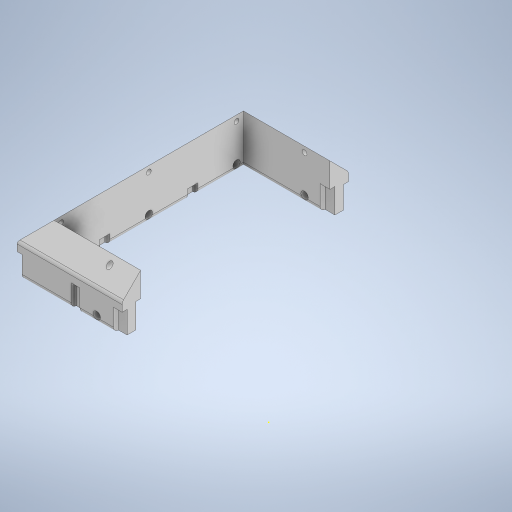
# Autodesk Inventor part: Palm_FingerAttachment
Saved by Autodesk Inventor 2023 (Build 270158000, 158)
## iProperties
Created: 2023-04-19
Part Number: Palm_FingerAttachment
Material: Generic
Document SubType Name: Modeling
Designer: 1senadi
Density: 1 g/cm^3
Appearance: Default
Author: 1senadi
Autodesk Inventor part; units mm, degrees
ref_plane "YZ Plane" through (0, 0, 0) normal (1, 0, 0) x (0, 1, 0)
ref_plane "XZ Plane" through (0, 0, 0) normal (0, 1, 0) x (-1, 0, 0)
ref_plane "XY Plane" through (0, 0, 0) normal (0, 0, 1) x (1, 0, 0)
sketch "Sketch1" plane through (0, 0, 0) normal (0, 1, 0) x (-1, 0, 0)
  line L0 (0, 0) -> (102, 0)
  line L1 (102, 0) -> (102, 91.8)
  line L2 (102, 91.8) -> (0, 91.8)
  line L3 (0, 91.8) -> (0, 0)
  line L4 (94.5, 84.3) -> (94.5, 7.5)
  line L5 (94.5, 7.5) -> (7.5, 7.5)
  line L6 (7.5, 7.5) -> (7.5, 84.3)
  line L7 (7.5, 84.3) -> (94.5, 84.3)
  dimension "d0" = 102
  dimension "d1" = 91.8
  dimension "d2" = 7.5
  constraints: 16 end point, 4 parallel, 2 perpendicular, 1 horizontal, 3 other
  measures "d0" distance of L2.end L1.end
  measures "d1" distance of L1.end L0.end
  measures "d2" distance between parallel lines of L1 L4
extrude "Extrusion1" add sketch "Sketch1" along normal blind 20
sketch "Sketch2" plane through (-102, 0, 0) normal (-1, 0, 0) x (0, 0, 1)
  line L0 (0, 0) -> (0, 9)
  line L1 (0, 0) -> (0, 20) projected
  line L2 (0, 9) -> (3.5, 9)
  line L3 (3.5, 9) -> (3.5, 0)
  line L4 (91.8, 0) -> (0, 0) projected
  line L5 (0, 0) -> (3.5, 0)
  line L6 (3.5, 0) -> (17.1, 0)
  line L7 (17.1, 0) -> (17.1, 9)
  line L8 (17.1, 9) -> (20.6, 9)
  line L9 (20.6, 9) -> (20.6, 0)
  line L10 (17.1, 0) -> (20.6, 0)
  line L11 (56.2, 9) -> (56.2, 0)
  line L12 (52.7, 9) -> (56.2, 9)
  line L13 (52.7, 0) -> (52.7, 9)
  line L14 (52.7, 0) -> (56.2, 0)
  line L15 (39.1, 0) -> (52.7, 0)
  line L16 (39.1, 9) -> (39.1, 0)
  line L17 (35.6, 9) -> (39.1, 9)
  line L18 (35.6, 0) -> (35.6, 9)
  line L19 (35.6, 0) -> (39.1, 0)
  line L20 (91.8, 9) -> (91.8, 0)
  line L21 (88.3, 9) -> (91.8, 9)
  line L22 (88.3, 0) -> (88.3, 9)
  line L23 (88.3, 0) -> (91.8, 0)
  line L24 (74.7, 0) -> (88.3, 0)
  line L25 (74.7, 9) -> (74.7, 0)
  line L26 (71.2, 9) -> (74.7, 9)
  line L27 (71.2, 0) -> (71.2, 9)
  line L28 (71.2, 0) -> (74.7, 0)
  point P0 (88.3, 0)
  point P1 (74.7, 0)
  point P2 (52.7, 0)
  point P3 (39.1, 0)
  dimension "d5" = 9
  dimension "d6" = 3.5
  dimension "d7" = 13.6
  dimension "d8" = 9
  dimension "d9" = 3.5
  dimension "d12" = 35.6
  constraints: 54 end point, 6 perpendicular, 4 point on line, 1 collinear, 1 horizontal, 34 other
  measures "d5" distance of L0.start L0.end
  measures "d6" distance of L0.end L2.end
  measures "d7" distance of L3.end L6.end
  measures "d8" distance of L6.end L7.end
  measures "d9" distance of L7.end L8.end
  measures "d12" distance of L8.end L11.start
extrude "Extrusion2" cut sketch "Sketch2" against normal blind 2
sketch "Sketch3" plane through (-102, 20, 91.8) normal (0, 0, 1) x (1, 0, 0)
  point P0 (102, -20)
sketch "Sketch4" plane through (-102, 20, 91.8) normal (0, 0, 1) x (1, 0, 0)
  line L0 (2, -20) -> (0, -20) projected
  line L1 (2, -20) -> (22, -20)
  line L2 (7.5, -20) -> (94.5, -20) projected
  line L3 (22, -20) -> (22, -11)
  line L4 (22, -11) -> (25.5, -11)
  line L5 (25.5, -11) -> (25.5, -20)
  line L6 (22, -20) -> (25.5, -20)
  line L7 (25.5, -20) -> (39.1, -20)
  line L8 (39.1, -20) -> (39.1, -11)
  line L9 (39.1, -11) -> (42.6, -11)
  line L10 (42.6, -11) -> (42.6, -20)
  line L11 (42.6, -20) -> (39.1, -20)
  point P0 (102, -20)
  dimension "d19" = 20
  dimension "d20" = 9
  dimension "d21" = 3.5
  dimension "d22" = 13.6
  dimension "d23" = 9
  dimension "d24" = 3.5
  constraints: 20 end point, 6 point on line, 3 perpendicular, 2 collinear, 1 vertical
  measures "d19" distance of L0.start L1.end
  measures "d20" distance of L1.end L3.end
  measures "d21" distance of L3.end L4.end
  measures "d22" distance of L5.end L7.end
  measures "d23" distance of L7.end L8.end
  measures "d24" distance of L8.end L9.end
extrude "Extrusion3" cut sketch "Sketch4" against normal blind 2
ref_plane "Work Plane1" through (-102, 0, 45.9) normal (0, 0, 1) x (1, 0, 0)
sketch "Sketch5" plane through (0, 0, 0) normal (0, -1, 0) x (1, 0, 0)
  line L0 (0, 0) -> (-100, 0) projected
  line L1 (0, 91.8) -> (0, 0) projected
  line L2 (-59.4, 91.8) -> (0, 91.8) projected
  line L3 (-59.4, 91.8) -> (-59.4, 89.8) projected
  line L4 (-59.4, 89.8) -> (-62.9, 89.8) projected
  line L5 (-62.9, 89.8) -> (-62.9, 91.8) projected
  line L6 (-76.5, 91.8) -> (-62.9, 91.8) projected
  line L7 (-76.5, 91.8) -> (-76.5, 89.8) projected
  line L8 (-76.5, 89.8) -> (-80, 89.8) projected
  line L9 (-80, 89.8) -> (-80, 91.8) projected
  line L10 (-100, 91.8) -> (-80, 91.8) projected
  line L11 (-100, 91.8) -> (-100, 88.3) projected
  line L12 (-100, 88.3) -> (-102, 88.3) projected
  line L13 (-102, 74.7) -> (-102, 88.3) projected
  line L14 (-102, 74.7) -> (-100, 74.7) projected
  line L15 (-100, 74.7) -> (-100, 71.2) projected
  line L16 (-100, 71.2) -> (-102, 71.2) projected
  line L17 (-102, 56.2) -> (-102, 71.2) projected
  line L18 (-102, 56.2) -> (-100, 56.2) projected
  line L19 (-100, 56.2) -> (-100, 52.7) projected
  line L20 (-100, 52.7) -> (-102, 52.7) projected
  line L21 (-102, 39.1) -> (-102, 52.7) projected
  line L22 (-102, 39.1) -> (-100, 39.1) projected
  line L23 (-100, 39.1) -> (-100, 35.6) projected
  line L24 (-100, 35.6) -> (-102, 35.6) projected
  line L25 (-102, 20.6) -> (-102, 35.6) projected
  line L26 (-102, 20.6) -> (-100, 20.6) projected
  line L27 (-100, 20.6) -> (-100, 17.1) projected
  line L28 (-100, 17.1) -> (-102, 17.1) projected
  line L29 (-102, 3.5) -> (-102, 17.1) projected
  line L30 (-102, 3.5) -> (-100, 3.5) projected
  line L31 (-100, 3.5) -> (-100, 0) projected
  line L32 (-94.5, 84.3) -> (-94.5, 7.5) projected
  line L33 (-7.5, 84.3) -> (-94.5, 84.3) projected
  line L34 (-7.5, 7.5) -> (-7.5, 84.3) projected
  line L35 (-94.5, 7.5) -> (-7.5, 7.5) projected
  line L36 (-59.4, 0) -> (-59.4, 2) projected
  line L37 (-59.4, 91.8) -> (-59.4, 89.8) projected
  line L38 (-59.4, 0) -> (-59.4, 91.8)
  line L39 (-102, 91.8) -> (0, 91.8) projected
  line L40 (-59.4, 91.8) -> (0, 91.8)
  line L41 (0, 91.8) -> (0, 0)
  line L42 (0, 0) -> (-102, 0) projected
  line L43 (-59.4, 0) -> (0, 0)
  point P0 (-80, 0)
  point P1 (-76.5, 0)
  point P2 (-62.9, 0)
  constraints: 8 end point, 1 collinear, 1 perpendicular
extrude "Extrusion4" cut sketch "Sketch5" against normal up to surface (20 mm away) contours L0 L36 L38 L35 L34 L33 L3 L2 L1 | L38 L33 L34 L35
sketch "Sketch6" plane through (-102, 9, 91.8) normal (0, 0, 1) x (1, 0, 0)
  line L0 (0, 11) -> (42.6, 11) projected
  line L1 (0, 11) -> (0, 3.5)
  line L2 (0, 0) -> (0, 11) projected
  line L3 (0, 3.5) -> (7.5, 11)
  line L4 (7.5, 11) -> (0, 11)
  point P0 (102, -9)
  point P1 (7.5, 11)
  dimension "d29" = 7.5
  dimension "d30" = 45
  constraints: 6 end point, 1 perpendicular, 1 point on line
  measures "d29" distance of L0.start L1.end
  measures "d30" angle of L3 L1
extrude "Extrusion5" cut sketch "Sketch6" against normal up to surface (91.8 mm away)
sketch "Sketch8" plane through (-102, 0, 20.6) normal (-1, 0, 0) x (0, 0, 1)
  line L0 (54.1, 0) -> (67.7, 0) projected
  line L1 (60.9, 0) -> (60.9, 2.75)
  line L2 (60.9, 0) -> (63.65, 0) construction
  circle A0 centre (60.9, 2.75) radius 1.5
  line L3 (60.9, 2.75) -> (60.9, 20)
  line L4 (-20.6, 20) -> (71.2, 20) projected
  line L5 (60.9, 20) -> (60.9, 17.75)
  circle A1 centre (60.9, 17.75) radius 1
  circle A2 centre (25.3, 2.75) radius 1.5
  circle A3 centre (25.3, 17.75) radius 1
  circle A4 centre (-10.3, 2.75) radius 1.5
  circle A5 centre (-10.3, 17.75) radius 1
  point P0 (-20.6, 0)
  point P1 (-13.1, 20)
  point P2 (63.7, 20)
  dimension "d38" = 2.75
  dimension "d39" = 90
  dimension "d40" = 3
  dimension "d41" = 2.25
  dimension "d42" = 2
  dimension "d45" = 35.6
  constraints: 8 end point, 6 centre point, 2 coincident, 2 horizontal, 2 point on line, 2 vertical, 1 midpoint, 1 perpendicular, 8 other
  measures "d38" distance of L1.start L1.end
  measures "d39" angle of L2 L1
  measures "d40" diameter of A0
  measures "d41" distance of L3.end L5.end
  measures "d42" diameter of A1
  measures "d45" distance of L3.start A2.centre
extrude "Extrusion7" cut sketch "Sketch8" against normal up to surface (7.5 mm away)
sketch "Sketch9" plane through (-102, 9, 91.8) normal (0, 0, 1) x (1, 0, 0)
  line L0 (25.5, -9) -> (39.1, -9) projected
  line L1 (32.3, -9) -> (32.3, -6.25)
  circle A0 centre (32.3, -6.25) radius 1.5
  line L2 (7.5, 11) -> (42.6, 11) projected
  line L3 (32.3, -9) -> (32.3, 11)
  line L4 (7.5, 11) -> (42.6, 11) projected
  line L5 (32.3, 11) -> (32.3, 8.75)
  circle A1 centre (32.3, 8.75) radius 1
  point P0 (102, -9)
  dimension "d52" = 2.75
  dimension "d53" = 3
  dimension "d54" = 2.25
  dimension "d55" = 2
  constraints: 6 end point, 2 centre point, 2 coincident, 2 point on line, 1 midpoint, 1 perpendicular, 1 vertical
  measures "d52" distance of L1.start L1.end
  measures "d53" diameter of A0
  measures "d54" distance of L3.end L5.end
  measures "d55" diameter of A1
extrude "Extrusion8" cut sketch "Sketch9" against normal up to surface (7.5 mm away)
mirror "Mirror2" about plane through (-102, 0, 45.9) normal (0, 0, 1) of "Extrusion8", "Extrusion3"
sketch "Sketch10" plane through (-59.4, 0, 89.8) normal (1, 0, 0) x (0, 0, -1)
  line L0 (-2, 9) -> (-2, 20) projected
  line L1 (-2, 20) -> (-2, 12.5)
  line L2 (-2, 20) -> (5.5, 20) construction
  line L3 (-2, 12.5) -> (5.5, 20)
  line L4 (89.8, 20) -> (-2, 20) projected
  line L5 (5.5, 20) -> (-2, 20)
  line L6 (89.8, 12.5) -> (89.8, 20) projected
  line L7 (89.8, 20) -> (89.8, 12.5)
  line L8 (89.8, 12.5) -> (82.3, 20)
  line L9 (82.3, 20) -> (89.8, 20)
  point P0 (89.8, 0)
  dimension "d58" = 7.5
  dimension "d59" = 90
  dimension "d60" = 45
  dimension "d61" = 45
  constraints: 14 end point, 4 collinear, 2 point on line, 1 horizontal, 1 perpendicular
  measures "d58" distance of L0.end L1.end
  measures "d59" angle of L1 L2
  measures "d60" angle of L3 L1
  measures "d61" angle of L7 L8
extrude "Extrusion9" cut sketch "Sketch10" against normal up to surface surface through (-94.5, 20, 91.8) normal (0.7071068, -0.7071068, 0)
sketch "Sketch11" plane through (-59.4, 0, 89.8) normal (1, 0, 0) x (0, 0, -1)
  line L0 (5.5, 0) -> (82.3, 0) projected
  line L1 (5.5, 0) -> (3.5, 0)
  line L2 (5.5, 0) -> (0, 0) projected
  line L3 (3.5, 0) -> (3.5, 10)
  line L4 (3.5, 10) -> (5.5, 10)
  line L5 (5.5, 0) -> (5.5, 20) projected
  line L6 (5.5, 0) -> (5.5, 10)
  line L7 (82.3, 0) -> (82.3, 20) projected
  line L8 (82.3, 0) -> (84.3, 0)
  line L9 (86.3, 0) -> (72.7, 0) projected
  line L10 (84.3, 0) -> (84.3, 10)
  line L11 (84.3, 10) -> (82.3, 10)
  line L12 (82.3, 10) -> (82.3, 0)
  point P0 (89.8, 0)
  dimension "d64" = 2
  dimension "d65" = 10
  dimension "d66" = 2
  dimension "d67" = 10
  dimension "d68" = 2
  constraints: 16 end point, 2 midpoint, 2 perpendicular, 2 point on line, 1 collinear
  measures "d64" distance of L0.start L1.end
  measures "d65" distance of L1.end L3.end
  measures "d66" distance of L0.end L8.end
  measures "d67" distance of L8.end L10.end
  measures "d68" distance of L10.end L11.end
extrude "Extrusion10" cut sketch "Sketch11" against normal blind 4
sketch "Sketch12" plane through (0, 0, 0) normal (0, -1, 0) x (1, 0, 0)
  line L0 (-100, 20.6) -> (-100, 17.1) projected
  line L1 (-100, 39.1) -> (-100, 35.6) projected
  line L2 (-100, 20.6) -> (-100, 35.6)
  line L3 (-100, 35.6) -> (-94.5, 35.6)
  line L4 (-94.5, 84.3) -> (-94.5, 7.5) projected
  line L5 (-100, 28.1) -> (-94.5, 28.1)
  line L6 (-94.5, 28.1) -> (-94.5, 26.1)
  line L7 (-94.5, 28.1) -> (-94.5, 30.1)
  line L8 (-94.5, 30.1) -> (-96.5, 30.1)
  line L9 (-96.5, 30.1) -> (-96.5, 26.1)
  line L10 (-96.5, 26.1) -> (-94.5, 26.1)
  line L11 (-96.5, 61.7) -> (-94.5, 61.7)
  line L12 (-94.5, 63.7) -> (-94.5, 61.7)
  line L13 (-94.5, 63.7) -> (-94.5, 65.7)
  line L14 (-94.5, 65.7) -> (-96.5, 65.7)
  line L15 (-96.5, 65.7) -> (-96.5, 61.7)
  point P0 (0, 0)
  dimension "d71" = 2
  dimension "d72" = 2
  dimension "d73" = 2
  dimension "d76" = 35.6
  constraints: 26 end point, 4 perpendicular, 4 point on line, 2 vertical, 1 midpoint, 1 parallel, 10 other
  measures "d71" distance of L5.end L6.end
  measures "d72" distance of L5.end L7.end
  measures "d73" distance of L7.end L8.end
  measures "d76" distance of L9.end L11.start
extrude "Extrusion11" cut sketch "Sketch12" against normal blind 4 contours L9 L8 L4 L5 | L5 L4 L10 L9 | L4 L11 L15 L14
fillet "Fillet1" radius 2 5 edges at (-94.5, 0, 45.9) (-94.5, 0, 75) (-94.5, 0, 16.8) (-78.95, 0, 7.5) (-78.95, 0, 84.3)
fillet "Fillet2" radius 2 12 edges at (-69.7, 0, 0) (-90, 0, 0) (-102, 0, 10.3) (-102, 0, 28.1) (-102, 0, 45.9) (-102, 0, 63.7) (-102, 0, 81.5) (-90, 0, 91.8) (-69.7, 0, 91.8) (-102, 12.5, 45.9) (-80.7, 12.5, 91.8) (-80.7, 12.5, 0)
body "Solid1"
